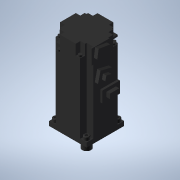
# Autodesk Inventor part: ETH2-17-M40B_8
Saved by Autodesk Inventor 2021 (Build 250183000, 183)
## iProperties
Created: 2025-05-01
Part Number: ETH2-17-M40B_8
Material: Generic
Catalog Web Link: www.cadenas.de
Description: ETH2_17_8-ETH2
Vendor: TOYO
Document SubType Name: Modeling
Designer: psAdmin
Manufacturer: TOYO
Mass: 445.454 g
Surface Area: 437.943 cm^2
Volume: 445.454 cm^3
Density: 1 g/cm^3
Appearance: PSOLRGB-175-175-175
Category: PARTsolutions
Company: TOYO
Title: ETH2-17-M40B
Author: Cadenas PARTsolutions
Comments: ETH2
PSOL_IDENT_0: {$CADENAS_DATA/23d-libs/toyo/eth2_series/eth2_17/parts/eth2_17_body8.prj},177 {VTYP=3D},{NB=ETH2-17-
PSOL_IDENT_1: M40B_8},{LINA=ETH2-17-M40B},{NN=ETH2_17_8},{DATE=02.07.2024 05:59:00},{GEOMDATE=05.06.2024 05:55:02}
PSOL_IDENT_2: ,{VERSION=},{LINEID=10},{WBVAR=MB,BRAKE},{WBNUMERIC=}  {NB=ETH2-17-M40B_8},{LINA=ETH2-17-M40B},{KT=D
PSOL_IDENT_3: UMMY},{CNSORDERNO=ETH2-17-M40B},{MODEL=ETH2-17},{MB=M},{POWEWR=40：400W},{BRAKE=B},{MBCODE=M40B}
NB: ETH2-17-M40B_8
NN: ETH2_17_8
NT: ETH2
NBSYN: $CNSORDERNO._8
LINA: ETH2-17-M40B
CATALOG: TOYO
MODEL: ETH2-17
MB: M:Mitsubishi
POWEWR: 40：400W
BRAKE: B:With brake
SUPPLIER: TOYO
ARTICLENO: ETH2-17-M40B_8
BOMINFO: ETH2-17-M40B
CREATOR: CADENAS GmbH
Autodesk Inventor part; units mm, degrees
sketch "Sketch_1" plane through (0, 0, 0) normal (0, 1, 0) x (-1, 0, 0)
  line L0 (30, 30) -> (-30, 30)
  line L1 (-30, 30) -> (-30, -30)
  line L2 (-30, -30) -> (30, -30)
  line L3 (30, -30) -> (30, 30)
  constraints: 8 end point
extrude "Extrusion1" add sketch "Sketch_1" along normal blind 114
sketch "Sketch_2" plane through (0, 114, 0) normal (0, 1, 0) x (1, 0, 0)
  line L0 (-29.95, -29.95) -> (29.95, -29.95)
  line L1 (29.95, -29.95) -> (29.95, 29.95)
  line L2 (29.95, 29.95) -> (-29.95, 29.95)
  line L3 (-29.95, 29.95) -> (-29.95, -29.95)
  constraints: 8 end point
extrude "Extrusion2" add sketch "Sketch_2" along normal blind 21.1
sketch "Sketch_3" plane through (0, 7, 0) normal (0, 1, 0) x (1, 0, 0)
  line L0 (-50, -50) -> (50, -50)
  line L1 (50, -50) -> (50, 50)
  line L2 (50, 50) -> (-50, 50)
  line L3 (-50, 50) -> (-50, -50)
  line L4 (-30, -19.5147) -> (-20.2, -20.2)
  line L5 (-20.2, -20.2) -> (-19.5147, -30)
  line L6 (-19.5147, -30) -> (19.5147, -30)
  line L7 (19.5147, -30) -> (20.2, -20.2)
  line L8 (20.2, -20.2) -> (30, -19.5147)
  line L9 (30, -19.5147) -> (30, 19.5147)
  line L10 (30, 19.5147) -> (20.2, 20.2)
  line L11 (20.2, 20.2) -> (19.5147, 30)
  line L12 (19.5147, 30) -> (-19.5147, 30)
  line L13 (-19.5147, 30) -> (-20.2, 20.2)
  line L14 (-20.2, 20.2) -> (-30, 19.5147)
  line L15 (-30, 19.5147) -> (-30, -19.5147)
  constraints: 32 end point
extrude "Extrusion3" cut sketch "Sketch_3" along normal blind 141.9
sketch "Sketch_4" plane through (0, 110, 0) normal (0, 1, 0) x (1, 0, 0)
  line L0 (-22.8, -33) -> (-12.8, -33)
  line L1 (-12.8, -33) -> (-12.8, -23)
  line L2 (-12.8, -23) -> (-22.8, -23)
  line L3 (-22.8, -23) -> (-22.8, -33)
  constraints: 8 end point
extrude "Extrusion4" cut sketch "Sketch_4" along normal blind 8.5
sketch "Sketch_24" plane through (0, 110, 0) normal (0, 1, 0) x (1, 0, 0)
  line L0 (-33, 22.8) -> (-33, 12.8)
  line L1 (-33, 12.8) -> (-23, 12.8)
  line L2 (-23, 12.8) -> (-23, 22.8)
  line L3 (-23, 22.8) -> (-33, 22.8)
  constraints: 8 end point
extrude "Extrusion5" cut sketch "Sketch_24" along normal blind 8.5
sketch "Sketch_5" plane through (0, 110, 0) normal (0, 1, 0) x (1, 0, 0)
  line L0 (12.8, 33) -> (12.8, 23)
  line L1 (12.8, 23) -> (22.8, 23)
  line L2 (22.8, 23) -> (22.8, 33)
  line L3 (22.8, 33) -> (12.8, 33)
  constraints: 8 end point
extrude "Extrusion6" cut sketch "Sketch_5" along normal blind 8.5
sketch "Sketch_6" plane through (0, 118.5, 0) normal (0, 1, 0) x (1, 0, 0)
  line L0 (-32.5, -22.5) -> (-22.5, -22.5)
  line L1 (-22.5, -22.5) -> (-22.5, -12.5)
  line L2 (-22.5, -12.5) -> (-32.5, -12.5)
  line L3 (-32.5, -12.5) -> (-32.5, -22.5)
  constraints: 8 end point
extrude "Extrusion7" cut sketch "Sketch_6" along normal blind 30
sketch "Sketch_7" plane through (0, 118.5, 0) normal (0, 1, 0) x (1, 0, 0)
  line L0 (22.5, 22.5) -> (22.5, 12.5)
  line L1 (22.5, 12.5) -> (32.5, 12.5)
  line L2 (32.5, 12.5) -> (32.5, 22.5)
  line L3 (32.5, 22.5) -> (22.5, 22.5)
  constraints: 8 end point
extrude "Extrusion8" cut sketch "Sketch_7" along normal blind 30
sketch "Sketch_8" plane through (0, 118.5, 0) normal (0, 1, 0) x (1, 0, 0)
  line L0 (12.5, -32.5) -> (22.5, -32.5)
  line L1 (22.5, -32.5) -> (22.5, -22.5)
  line L2 (22.5, -22.5) -> (12.5, -22.5)
  line L3 (12.5, -22.5) -> (12.5, -32.5)
  constraints: 8 end point
extrude "Extrusion9" cut sketch "Sketch_8" along normal blind 30
sketch "Sketch_9" plane through (0, 118.5, 0) normal (0, 1, 0) x (1, 0, 0)
  line L0 (-22.5, 32.5) -> (-22.5, 22.5)
  line L1 (-22.5, 22.5) -> (-12.5, 22.5)
  line L2 (-12.5, 22.5) -> (-12.5, 32.5)
  line L3 (-12.5, 32.5) -> (-22.5, 32.5)
  constraints: 8 end point
extrude "Extrusion10" cut sketch "Sketch_9" along normal blind 30
sketch "Sketch_10" plane through (0, 121.5, 0) normal (0, 1, 0) x (1, 0, 0)
  line L0 (-22.8, -33) -> (-12.8, -33)
  line L1 (-12.8, -33) -> (-12.8, -23)
  line L2 (-12.8, -23) -> (-22.8, -23)
  line L3 (-22.8, -23) -> (-22.8, -33)
  constraints: 8 end point
extrude "Extrusion11" cut sketch "Sketch_10" along normal blind 30
sketch "Sketch_25" plane through (0, 121.5, 0) normal (0, 1, 0) x (1, 0, 0)
  line L0 (-33, 22.8) -> (-33, 12.8)
  line L1 (-33, 12.8) -> (-23, 12.8)
  line L2 (-23, 12.8) -> (-23, 22.8)
  line L3 (-23, 22.8) -> (-33, 22.8)
  constraints: 8 end point
extrude "Extrusion12" cut sketch "Sketch_25" along normal blind 20
sketch "Sketch_11" plane through (0, 121.5, 0) normal (0, 1, 0) x (1, 0, 0)
  line L0 (12.8, 33) -> (12.8, 23)
  line L1 (12.8, 23) -> (22.8, 23)
  line L2 (22.8, 23) -> (22.8, 33)
  line L3 (22.8, 33) -> (12.8, 33)
  constraints: 8 end point
extrude "Extrusion13" cut sketch "Sketch_11" along normal blind 30
sketch "Sketch_12" plane through (16.3, 0, 0) normal (1, 0, 0) x (0, 0, -1)
  line L0 (-26.5, 121.1) -> (-26.5, 118.5)
  line L1 (-26.5, 118.5) -> (-29.25, 118.5)
  line L2 (-29.25, 118.5) -> (-29.25, 121.1)
  line L3 (-29.25, 121.1) -> (-26.5, 121.1)
  line L4 (-26.5, 121.1) -> (-26.5, 118.5)
  constraints: 10 end point
revolve "Revolution1" add sketch "Sketch_12" angle 360 about axis through (16.3, 121.1, 26.5) along (0, 1, 0)
sketch "Sketch_13" plane through (-16.3, 0, 0) normal (1, 0, 0) x (0, 0, -1)
  line L0 (26.5, 121.1) -> (26.5, 118.5)
  line L1 (26.5, 118.5) -> (23.75, 118.5)
  line L2 (23.75, 118.5) -> (23.75, 121.1)
  line L3 (23.75, 121.1) -> (26.5, 121.1)
  line L4 (26.5, 121.1) -> (26.5, 118.5)
  constraints: 10 end point
revolve "Revolution2" add sketch "Sketch_13" angle 360 about axis through (-16.3, 121.1, -26.5) along (0, 1, 0)
sketch "Sketch_14" plane through (16.66, 0, 0) normal (1, 0, 0) x (0, 0, -1)
  line L0 (27.0849, 110) -> (27.0849, 112.6)
  line L1 (27.0849, 112.6) -> (29.8349, 112.6)
  line L2 (29.8349, 112.6) -> (29.8349, 110)
  line L3 (29.8349, 110) -> (27.0849, 110)
  line L4 (27.0849, 110) -> (27.0849, 112.6)
  constraints: 10 end point
revolve "Revolution3" add sketch "Sketch_14" angle 360 about axis through (16.66, 110, -27.0849) along (0, -1, 0)
sketch "Sketch_15" plane through (-16.66, 0, 0) normal (1, 0, 0) x (0, 0, -1)
  line L0 (-27.0849, 110) -> (-27.0849, 112.6)
  line L1 (-27.0849, 112.6) -> (-24.3349, 112.6)
  line L2 (-24.3349, 112.6) -> (-24.3349, 110)
  line L3 (-24.3349, 110) -> (-27.0849, 110)
  line L4 (-27.0849, 110) -> (-27.0849, 112.6)
  constraints: 10 end point
revolve "Revolution4" add sketch "Sketch_15" angle 360 about axis through (-16.66, 110, 27.0849) along (0, -1, 0)
sketch "Sketch_16" plane through (0, 0, 16.3) normal (0, 0, 1) x (1, 0, 0)
  line L0 (-26.5, 118.5) -> (-26.5, 121.1)
  line L1 (-26.5, 121.1) -> (-23.75, 121.1)
  line L2 (-23.75, 121.1) -> (-23.75, 118.5)
  line L3 (-23.75, 118.5) -> (-26.5, 118.5)
  line L4 (-26.5, 118.5) -> (-26.5, 121.1)
  constraints: 10 end point
revolve "Revolution5" add sketch "Sketch_16" angle 360 about axis through (-26.5, 118.5, 16.3) along (0, -1, 0)
sketch "Sketch_17" plane through (0, 0, -16.3) normal (0, 0, 1) x (1, 0, 0)
  line L0 (26.5, 118.5) -> (26.5, 121.1)
  line L1 (26.5, 121.1) -> (29.25, 121.1)
  line L2 (29.25, 121.1) -> (29.25, 118.5)
  line L3 (29.25, 118.5) -> (26.5, 118.5)
  line L4 (26.5, 118.5) -> (26.5, 121.1)
  constraints: 10 end point
revolve "Revolution6" add sketch "Sketch_17" angle 360 about axis through (26.5, 118.5, -16.3) along (0, -1, 0)
sketch "Sketch_26" plane through (0, 0, -16.66) normal (0, 0, 1) x (1, 0, 0)
  line L0 (-27.0849, 110) -> (-27.0849, 112.6)
  line L1 (-27.0849, 112.6) -> (-24.3349, 112.6)
  line L2 (-24.3349, 112.6) -> (-24.3349, 110)
  line L3 (-24.3349, 110) -> (-27.0849, 110)
  line L4 (-27.0849, 110) -> (-27.0849, 112.6)
  constraints: 10 end point
revolve "Revolution7" add sketch "Sketch_26" angle 360 about axis through (-27.0849, 110, -16.66) along (0, -1, 0)
sketch "Sketch_18" plane through (0, 114, 0) normal (0, 1, 0) x (1, 0, 0)
  line L0 (21.95, -18.0392) -> (21.95, -20.0392)
  line L1 (21.95, -20.0392) -> (29.95, -20.0392)
  line L2 (29.95, -20.0392) -> (29.95, -18.0392)
  line L3 (29.95, -18.0392) -> (21.95, -18.0392)
  constraints: 8 end point
extrude "Extrusion14" add sketch "Sketch_18" along normal blind 21.1
sketch "Sketch_19" plane through (29.95, 0, 0) normal (1, 0, 0) x (0, 0, -1)
  line L0 (-23.7, 135.1) -> (-23.7, 111.6)
  line L1 (-23.7, 111.6) -> (4.7, 111.6)
  line L2 (4.7, 111.6) -> (4.7, 135.1)
  line L3 (4.7, 135.1) -> (-23.7, 135.1)
  constraints: 8 end point
extrude "Extrusion15" add sketch "Sketch_19" along normal blind 2.05
sketch "Sketch_20" plane through (29.95, 0, 0) normal (1, 0, 0) x (0, 0, -1)
  line L0 (-20.4781, 120.7723) -> (-1.712, 117.8)
  line L1 (-1.712, 117.8) -> (0.4781, 131.6276)
  line L2 (0.4781, 131.6276) -> (-18.288, 134.5999)
  line L3 (-18.288, 134.5999) -> (-20.4781, 120.7723)
  constraints: 8 end point
extrude "Extrusion16" add sketch "Sketch_20" along normal blind 7.55
sketch "Sketch_21" plane through (30, 0, 0) normal (1, 0, 0) x (0, 0, -1)
  line L0 (-8, 69.85) -> (-8, 51.7)
  line L1 (-8, 51.7) -> (19.8, 51.7)
  line L2 (19.8, 51.7) -> (19.8, 69.85)
  line L3 (19.8, 69.85) -> (-8, 69.85)
  constraints: 8 end point
extrude "Extrusion17" add sketch "Sketch_21" along normal blind 3.4
sketch "Sketch_22" plane through (30, 0, 0) normal (1, 0, 0) x (0, 0, -1)
  line L0 (-1.65, 64.925) -> (-1.65, 57.475)
  line L1 (-1.65, 57.475) -> (13.45, 57.475)
  line L2 (13.45, 57.475) -> (13.45, 64.925)
  line L3 (13.45, 64.925) -> (-1.65, 64.925)
  constraints: 8 end point
extrude "Extrusion18" add sketch "Sketch_22" along normal blind 8.8
sketch "Sketch_27" plane through (30, 0, 0) normal (1, 0, 0) x (0, 0, -1)
  line L0 (-17.0218, 84.1526) -> (1.4532, 79.7171)
  line L1 (1.4532, 79.7171) -> (5.4218, 96.2474)
  line L2 (5.4218, 96.2474) -> (-13.0532, 100.6829)
  line L3 (-13.0532, 100.6829) -> (-17.0218, 84.1526)
  constraints: 8 end point
extrude "Extrusion19" add sketch "Sketch_27" along normal blind 5.3
sketch "Sketch_28" plane through (30, 0, 0) normal (1, 0, 0) x (0, 0, -1)
  line L0 (-10.8994, 87.5934) -> (-2.4398, 85.5624)
  line L1 (-2.4398, 85.5624) -> (-0.7006, 92.8066)
  line L2 (-0.7006, 92.8066) -> (-9.1602, 94.8376)
  line L3 (-9.1602, 94.8376) -> (-10.8994, 87.5934)
  constraints: 8 end point
extrude "Extrusion20" add sketch "Sketch_28" along normal blind 10.8
sketch "Sketch_23" plane through (0, 0, 0) normal (0, 0, 1) x (1, 0, 0)
  line L0 (0, -30) -> (0, 0)
  line L1 (0, 0) -> (25, 0)
  line L2 (25, 0) -> (25, -3)
  line L3 (25, -3) -> (7, -3)
  line L4 (7, -3) -> (7, -30)
  line L5 (7, -30) -> (0, -30)
  line L6 (0, -30) -> (0, 0)
  constraints: 14 end point
revolve "Revolution8" add sketch "Sketch_23" angle 360 about axis through (0, -30, 0) along (0, -1, 0)
sketch "Sketch_29" plane through (0, 0, 0) normal (0.7071068, 0, 0.7071068) x (0.7071068, 0, -0.7071068)
  line L0 (35, 0) -> (35, 12)
  line L1 (35, 12) -> (38.75, 12)
  line L2 (38.75, 12) -> (39.25, 11.5)
  line L3 (39.25, 11.5) -> (39.25, 7)
  line L4 (39.25, 7) -> (37, 7)
  line L5 (37, 7) -> (37, 0)
  line L6 (37, 0) -> (35, 0)
  line L7 (35, 0) -> (35, 12)
  constraints: 16 end point
revolve "Revolution9" add sketch "Sketch_29" angle 360 about axis through (24.7487, 0, -24.7487) along (0, -1, 0)
sketch "Sketch_30" plane through (0, 0, 0) normal (0.7071068, 0, 0.7071068) x (0.7071068, 0, -0.7071068)
  line L0 (-35, 0) -> (-35, 12)
  line L1 (-35, 12) -> (-31.25, 12)
  line L2 (-31.25, 12) -> (-30.75, 11.5)
  line L3 (-30.75, 11.5) -> (-30.75, 7)
  line L4 (-30.75, 7) -> (-33, 7)
  line L5 (-33, 7) -> (-33, 0)
  line L6 (-33, 0) -> (-35, 0)
  line L7 (-35, 0) -> (-35, 12)
  constraints: 16 end point
revolve "Revolution10" add sketch "Sketch_30" angle 360 about axis through (-24.7487, 0, 24.7487) along (0, -1, 0)
sketch "Sketch_31" plane through (0, 0, 0) normal (-0.7071068, 0, 0.7071068) x (0.7071068, 0, 0.7071068)
  line L0 (35, 0) -> (35, 12)
  line L1 (35, 12) -> (38.75, 12)
  line L2 (38.75, 12) -> (39.25, 11.5)
  line L3 (39.25, 11.5) -> (39.25, 7)
  line L4 (39.25, 7) -> (37, 7)
  line L5 (37, 7) -> (37, 0)
  line L6 (37, 0) -> (35, 0)
  line L7 (35, 0) -> (35, 12)
  constraints: 16 end point
revolve "Revolution11" add sketch "Sketch_31" angle 360 about axis through (24.7487, 0, 24.7487) along (0, -1, 0)
sketch "Sketch_32" plane through (0, 0, 0) normal (-0.7071068, 0, 0.7071068) x (0.7071068, 0, 0.7071068)
  line L0 (-35, 0) -> (-35, 12)
  line L1 (-35, 12) -> (-31.25, 12)
  line L2 (-31.25, 12) -> (-30.75, 11.5)
  line L3 (-30.75, 11.5) -> (-30.75, 7)
  line L4 (-30.75, 7) -> (-33, 7)
  line L5 (-33, 7) -> (-33, 0)
  line L6 (-33, 0) -> (-35, 0)
  line L7 (-35, 0) -> (-35, 12)
  constraints: 16 end point
revolve "Revolution12" add sketch "Sketch_32" angle 360 about axis through (-24.7487, 0, -24.7487) along (0, -1, 0)
sketch "Sketch_33" plane through (0, 12, 0) normal (0, 1, 0) x (1, 0, 0)
  line L0 (22.7487, -25.9034) -> (24.7487, -27.0581)
  line L1 (24.7487, -27.0581) -> (26.7487, -25.9034)
  line L2 (26.7487, -25.9034) -> (26.7487, -23.594)
  line L3 (26.7487, -23.594) -> (24.7487, -22.4393)
  line L4 (24.7487, -22.4393) -> (22.7487, -23.594)
  line L5 (22.7487, -23.594) -> (22.7487, -25.9034)
  constraints: 12 end point
extrude "Extrusion21" cut sketch "Sketch_33" against normal blind 2.5
sketch "Sketch_34" plane through (0, 12, 0) normal (0, 1, 0) x (1, 0, 0)
  line L0 (22.7487, 23.594) -> (24.7487, 22.4393)
  line L1 (24.7487, 22.4393) -> (26.7487, 23.594)
  line L2 (26.7487, 23.594) -> (26.7487, 25.9034)
  line L3 (26.7487, 25.9034) -> (24.7487, 27.0581)
  line L4 (24.7487, 27.0581) -> (22.7487, 25.9034)
  line L5 (22.7487, 25.9034) -> (22.7487, 23.594)
  constraints: 12 end point
extrude "Extrusion22" cut sketch "Sketch_34" against normal blind 2.5
sketch "Sketch_35" plane through (0, 12, 0) normal (0, 1, 0) x (1, 0, 0)
  line L0 (-26.7487, 23.594) -> (-24.7487, 22.4393)
  line L1 (-24.7487, 22.4393) -> (-22.7487, 23.594)
  line L2 (-22.7487, 23.594) -> (-22.7487, 25.9034)
  line L3 (-22.7487, 25.9034) -> (-24.7487, 27.0581)
  line L4 (-24.7487, 27.0581) -> (-26.7487, 25.9034)
  line L5 (-26.7487, 25.9034) -> (-26.7487, 23.594)
  constraints: 12 end point
extrude "Extrusion23" cut sketch "Sketch_35" against normal blind 2.5
sketch "Sketch_36" plane through (0, 12, 0) normal (0, 1, 0) x (1, 0, 0)
  line L0 (-26.7487, -25.9034) -> (-24.7487, -27.0581)
  line L1 (-24.7487, -27.0581) -> (-22.7487, -25.9034)
  line L2 (-22.7487, -25.9034) -> (-22.7487, -23.594)
  line L3 (-22.7487, -23.594) -> (-24.7487, -22.4393)
  line L4 (-24.7487, -22.4393) -> (-26.7487, -23.594)
  line L5 (-26.7487, -23.594) -> (-26.7487, -25.9034)
  constraints: 12 end point
extrude "Extrusion24" cut sketch "Sketch_36" against normal blind 2.5
ref_plane "m_d_XY" through (0, 0, 0) normal (0, 1, 0) x (1, 0, 0)
ref_plane "m_d_YZ" through (0, 0, 0) normal (1, 0, 0) x (0, 0, -1)
ref_plane "m_d_ZX" through (0, 0, 0) normal (0, 0, -1) x (0, 1, 0)
body "Solid1"
